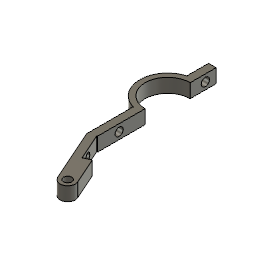
Trumpet+Clamp+3+Main (Autodesk Fusion 360 design; units mm, degrees)
Autodesk Fusion 360 part; units mm, degrees
sketch "Sketch1" plane through (0, 0, 0) normal (0, 1, 0) x (1, 0, 0)
  circle A0 centre (0, 0) radius 12.435
  circle A1 centre (0, 0) radius 15.435
  line L0 (0, 0) -> (-15.435, 0) construction
  line L1 (0, 0) -> (15.435, 0) construction
  line L2 (-4.25, -40.647) -> (8.6182, -69.5153)
  line L3 (4.25, -38.8384) -> (16.3818, -66.0547)
  circle A2 centre (12.5, -67.785) radius 4.25
  line L4 (12.5, -67.785) -> (8.6182, -69.5153) construction
  line L5 (12.5, -67.785) -> (16.3818, -66.0547) construction
  circle A3 centre (12.5, -67.785) radius 2.25
  line L6 (-4.25, -40.647) -> (-4.25, -14.8384)
  line L7 (4.25, -38.8384) -> (4.25, -14.8384)
  line L8 (0, 0) -> (0, -38.8384) construction
  line L9 (4.25, -38.8384) -> (-4.25, -38.8384) construction
  line L10 (-4.25, 14.8384) -> (-4.25, 26.8384)
  line L11 (-4.25, 26.8384) -> (4.25, 26.8384)
  line L12 (4.25, 26.8384) -> (4.25, 14.8384)
  line L13 (-4.25, 14.8384) -> (-4.25, -14.8384) construction
  line L14 (4.25, -14.8384) -> (4.25, 14.8384) construction
  line L15 (12.5, -67.785) -> (12.5, -72.035) construction
  point P0 (0, -15.435)
  dimension "d1" = 24.87
  dimension "d3" = 4.5
  dimension "d4" = 8.5
  dimension "d5" = 12.5
  dimension "d19" = 8.5
  dimension "d22" = 30.87
  dimension "d27" = 24
  dimension "d28" = 12
  dimension "d32" = 56.6
  constraint coincident A0.centre A1.centre
  constraint concentric A0 A1
  constraint coincident A1 L0.end
  constraint horizontal L0
  constraint coincident A1 L1.end
  constraint parallel L0 L1
  constraint coincident A2.centre L4.start
  constraint coincident A2 L2.end
  constraint coincident A2 L3.end
  constraint parallel L4 L5
  constraint coincident L2.end L4.end
  constraint coincident L3.end L5.end
  constraint coincident A1 L6.end
  constraint coincident A1 L7.end
  constraint parallel L2 L3
  constraint vertical L6
  constraint vertical L7
  constraint vertical L8
  constraint tangent L3 A2
  constraint coincident L6 L9.end
  constraint perpendicular L6 L9
  constraint midpoint L8.end L9
  constraint coincident A1 L10.start
  constraint vertical L10
  constraint perpendicular L10 L11
  constraint coincident A1 L12.end
  constraint perpendicular L11 L12
  constraint vertical L13
  constraint vertical L14
  constraint coincident A2 L15.end
  constraint vertical L15
  constraint coincident A1 P0
  constraint coincident L8 P0
  measures "d1" diameter of A0
  measures "d3" diameter of A3
  measures "d4" diameter of A2
  measures "d5" horizontal distance of A0.centre A2.centre
  measures "d19" distance of L6 L7
  measures "d22" diameter of A1
  measures "d27" distance of L3.start L7.end
  measures "d28" distance of L11.end L12.end
  measures "d32" vertical distance of L15.end P0
extrude "Extrude1" add sketch "Sketch1" along normal blind 7.7
sketch "Sketch2" plane through (-10.8972, 0, 4.8575) normal (0.913367, 0, -0.407138) x (-0.407138, 0, -0.913367)
  line L0 (-67.0018, 0) -> (-37.204, 0)
  line L1 (-37.204, 0) -> (-37.204, 7.7)
  line L2 (-37.204, 7.7) -> (-67.0018, 7.7)
  line L3 (-67.0018, 7.7) -> (-67.0018, 0)
  line L4 (-37.204, 3.85) -> (-67.0018, 3.85) construction
  circle A0 centre (-45.204, 3.85) radius 2.25
  dimension "d29" = 8
  dimension "d30" = 4.5
  constraint midpoint L1 L4.start
  constraint midpoint L3 L4.end
  constraint coincident L4 A0.centre
  measures "d29" distance of L4.start A0.centre
  measures "d30" diameter of A0
extrude "Extrude2" cut sketch "Sketch2" against normal up to surface (8.5 mm away) contours A0
sketch "Sketch3" plane through (4.25, 0, 0) normal (1, 0, 0) x (0, 0, -1)
  line L0 (-38.8384, 0) -> (-14.8384, 0)
  line L1 (-14.8384, 0) -> (-14.8384, 7.7)
  line L2 (-14.8384, 7.7) -> (-38.8384, 7.7)
  line L3 (-38.8384, 7.7) -> (-38.8384, 0)
  line L4 (-14.8384, 3.85) -> (-38.8384, 3.85) construction
  circle A0 centre (-26.8384, 3.85) radius 2.25
  line L5 (14.8384, 0) -> (26.8384, 0)
  line L6 (26.8384, 0) -> (26.8384, 7.7)
  line L7 (26.8384, 7.7) -> (14.8384, 7.7)
  line L8 (14.8384, 7.7) -> (14.8384, 0)
  line L9 (14.8384, 3.85) -> (26.8384, 3.85) construction
  circle A1 centre (20.8384, 3.85) radius 2.25
  dimension "d16" = 4.5
  constraint midpoint L1 L4.start
  constraint midpoint L3 L4.end
  constraint midpoint L4 A0.centre
  constraint midpoint L8 L9.start
  constraint midpoint L6 L9.end
  constraint midpoint L9 A1.centre
  constraint equal A0 A1
  measures "d16" diameter of A0
extrude "Extrude3" cut sketch "Sketch3" against normal up to surface (8.5 mm away) contours A0 | A1
sketch "Sketch4" plane through (0, 0, 0) normal (1, 0, 0) x (0, 0, -1)
  line L0 (-38.8384, 0) -> (-14.8384, 0) construction
  line L1 (-14.8384, 0) -> (-14.8384, 7.7) construction
  line L2 (-14.8384, 7.7) -> (-38.8384, 7.7) construction
  line L3 (-38.8384, 7.7) -> (-38.8384, 0) construction
  line L4 (14.8384, 0) -> (-14.8384, 0) construction
  line L5 (-14.8384, 0) -> (-14.8384, 7.7) construction
  line L6 (14.8384, 7.7) -> (-14.8384, 7.7) construction
  line L7 (-14.8384, 7.7) -> (-14.8384, 0) construction
  line L8 (-14.8384, 0) -> (-40.647, 0) construction
  line L9 (-40.647, 0) -> (-40.647, 7.7) construction
  line L10 (-40.647, 7.7) -> (-14.8384, 7.7) construction
  line L11 (-14.8384, 7.7) -> (-14.8384, 0) construction
  line L12 (14.8384, 0) -> (-39.7427, 0)
  line L13 (-39.7427, 0) -> (-39.7427, 7.7)
  line L14 (-39.7427, 7.7) -> (14.8384, 7.7)
  line L15 (14.8384, 7.7) -> (14.8384, 0)
  line L16 (-40.647, 7.7) -> (-38.8384, 7.7) construction
  line L17 (14.8384, 7.7) -> (14.8384, 0)
  line L18 (14.8384, 0) -> (-14.8384, 0)
  line L19 (14.8384, 0) -> (14.8384, 7.7)
  line L20 (14.8384, 7.7) -> (-14.8384, 7.7)
  circle A0 centre (20.8384, 3.85) radius 2.25
  line L21 (14.8384, 0) -> (26.8384, 0)
  line L22 (26.8384, 0) -> (26.8384, 7.7)
  line L23 (26.8384, 7.7) -> (14.8384, 7.7)
  line L24 (14.8384, 7.7) -> (14.8384, 0)
  circle A1 centre (-26.8384, 3.85) radius 2.25
  circle A2 centre (-26.8384, 3.85) radius 2.25
  constraint horizontal L12
  constraint vertical L13
  constraint horizontal L14
  constraint vertical L15
  constraint coincident L10 L13.end
  constraint coincident L4.start L12.start
  constraint coincident L9.end L10.start
  constraint coincident L2.end L3.start
  constraint midpoint L13.end L16
extrude "Extrude4" cut sketch "Sketch4" along normal blind 30 contours L12 L13 L14 L15 L17 L18 L19 L20 L24 | L15 L17 L19 L21 L22 L23 L24 | A1 A2
ref_plane "WorkPlane1" through (6.0659, 3.85, 53.3509) normal (-0.913367, 0, 0.407138) x (0.407138, 0, 0.913367)
sketch "Sketch5" plane through (-14.779, 0, 6.5878) normal (-0.913367, 0, 0.407138) x (0.407138, 0, 0.913367)
  circle A0 centre (45.204, 3.85) radius 2.25 construction
  line L0 (35.3953, 0) -> (67.0018, 0) construction
  line L1 (67.0018, 0) -> (67.0018, 7.7) construction
  line L2 (67.0018, 7.7) -> (35.3953, 7.7) construction
  line L3 (35.3953, 7.7) -> (35.3953, 0) construction
  line L4 (35.3953, 7.7) -> (51.1986, 7.7)
  line L5 (51.1986, 7.7) -> (51.1986, 0)
  line L6 (51.1986, 0) -> (35.3953, 0)
  line L7 (35.3953, 0) -> (35.3953, 7.7)
  constraint horizontal L4
  constraint vertical L5
  constraint horizontal L6
  constraint vertical L7
  constraint midpoint L0 L5.end
  constraint coincident L2.end L3.start
extrude "Extrude5" cut sketch "Sketch5" against normal up to surface (4.25 mm away)
equation "d19 = d4"
equation "d22 = d1 + 6 mm"
